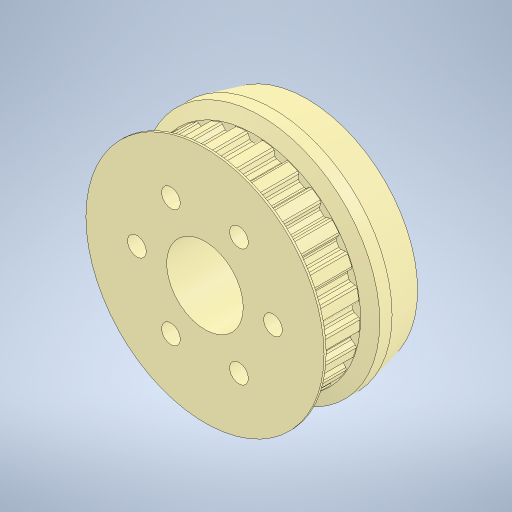
# Autodesk Inventor part: XL Belt Generator
Saved by Autodesk Inventor 2023.4 (Build 274418000, 418)
## iProperties
RuleStatus: InUse
Created: 2022-06-22
Part Number: XL Belt Generator
Material: Nylon 6/6
Document SubType Name: Modeling
Designer: Nathan Cai
Density: 1.13 g/cm^3
Appearance: Nylon 6
Mass: 24.0881 g
Surface Area: 78.8918 cm^2
Volume: 21.3169 cm^3
Author: Nathan Cai
Autodesk Inventor part; units mm, degrees
ref_plane "YZ Plane" through (0, 0, 0) normal (1, 0, 0) x (0, 1, 0)
ref_plane "XZ Plane" through (0, 0, 0) normal (0, 1, 0) x (-1, 0, 0)
ref_plane "XY Plane" through (0, 0, 0) normal (0, 0, 1) x (1, 0, 0)
sketch "Sketch2" plane through (0, 0, 0) normal (0, 0, 1) x (1, 0, 0)
  circle A0 centre (0, 0) radius 20.2127 construction
  circle A1 centre (0, 0) radius 19.6977
  circle A2 centre (0, 0) radius 7.1437
  dimension "Pd" = 40.4254
  dimension "OD" = 39.3954
  dimension "d61" = 14.2875
  constraints: 3 centre point, 3 coincident
  measures "Pd" diameter of A0
  measures "OD" diameter of A1
  measures "d61" diameter of A2
extrude "Extrusion3" add sketch "Sketch2" along normal blind 7.62
sketch "Sketch3" plane through (0, 0, 7.62) normal (0, 0, 1) x (1, 0, 0)
  line L0 (0, 0) -> (0, 19.6977) construction
  circle A0 centre (0, 0) radius 19.6977 projected
  line L1 (0, 0) -> (4.8986, 19.0788) construction
  circle A1 centre (0, 0) radius 18.4277
  line L2 (0.811, 18.6413) -> (1.1735, 19.4185)
  line L3 (1.2841, 19.6558) -> (0, 0) construction
  arc A2 (1.5477, 19.6368) -> (1.1735, 19.4185) centre (1.5179, 19.258) ccw
  arc A3 (0.4572, 18.422) -> (0.811, 18.6413) centre (0.4666, 18.8019) ccw
  circle A4 centre (0, 0) radius 19.6977 projected
  line L4 (-0.811, 18.6413) -> (-1.1735, 19.4185)
  arc A5 (-1.1735, 19.4185) -> (-1.5477, 19.6368) centre (-1.5179, 19.258) ccw
  arc A6 (-0.811, 18.6413) -> (-0.4572, 18.422) centre (-0.4666, 18.8019) ccw
  point P0 (1.807, 18.3389)
  point P1 (1.5477, 19.6368)
  point P2 (-1.5477, 19.6368)
  dimension "d29" = 14.4
  dimension "d30" = 36.8554
  dimension "d31" = 25
  dimension "d33" = 3.738
  dimension "d34" = 0.76
  dimension "d35" = 0.76
  constraints: 14 point on circle, 10 end point, 6 symmetric about line, 5 centre point, 4 tangent, 1 coincident, 1 point on line, 1 vertical, 2 other
  measures "d29" angle of L0 L1
  measures "d30" diameter of A1
  measures "d31" angle of L0 L2
  measures "d33" angle of L0 L3
  measures "d34" diameter of A2
  measures "d35" diameter of A3
extrude "Extrusion4" cut sketch "Sketch3" against normal through all contours A2 L2 A3 A1 A6 L4 A5 A0 picked at (0.0508, 19.2696)
pattern_circular "Circular Pattern2" count 25 over 360 about axis through (0, 0, 0) along (0, 0, 1) of "Extrusion4"
ref_plane "Work Plane1" through (0, 0, 3.81) normal (0, 0, 1) x (1, 0, 0)
sketch "Sketch6" plane through (0, 0, 7.62) normal (0, 0, 1) x (1, 0, 0)
  circle A0 centre (0, 0) radius 22.225
  circle A1 centre (0, 0) radius 7.1437 projected
  dimension "d62" = 44.45
  constraints: 1 centre point, 1 coincident
  measures "d62" diameter of A0
extrude "Extrusion7" add sketch "Sketch6" along normal blind 1.5875
chamfer "Chamfer2" distance 1.1906 distance2 2.3813 1 edges at (-22.225, 0, 7.62) measured on face at (-22.225, 0, 8.12)
mirror "Mirror2" about plane through (0, 0, 3.81) normal (0, 0, 1) of "Extrusion7", "Chamfer2"
thicken "Thicken3" operation add thickness 1.905 both sides no extend neighbours no toward (0, 0, -1) faces at (16.9134, -2.3428, -1.5875)
thicken "Thicken4" operation add thickness 6.35 both sides no extend neighbours no toward (0, 0, -1) faces at (16.9134, -2.3428, -3.4925)
chamfer "Chamfer3" distance 6.35 distance2 1.5875 1 edges at (-22.225, 0, -9.8425) measured on face at (-22.225, 0, -9.3425)
sketch "Sketch7" plane through (0, 0, -9.8425) normal (0, 0, -1) x (-1, 0, 0)
  circle A0 centre (0, 0) radius 12.7 construction
  line L0 (0, 0) -> (12.7, 0) construction
  circle A1 centre (12.7, 0) radius 1.7526
  circle A2 centre (6.35, 10.9985) radius 1.7526
  circle A3 centre (-6.35, 10.9985) radius 1.7526
  circle A4 centre (-12.7, 0) radius 1.7526
  circle A5 centre (-6.35, -10.9985) radius 1.7526
  circle A6 centre (6.35, -10.9985) radius 1.7526
  dimension "d75" = 25.4
  dimension "d76" = 3.5052
  dimension "d79" = 360
  constraints: 6 centre point, 2 coincident, 2 end point, 1 horizontal, 1 horizontal alignment, 15 other
  measures "d76" diameter of A1
extrude "Extrusion8" cut sketch "Sketch7" against normal through all
equation "\"pitch\" = 5.08"
equation "\"width\" = 7.62"
equation "\"T_angle\" = 50deg"
equation "\"T_ht\" = 1.27"
equation "\"r1\" = 0.38"
equation "\"r2\" = 0.38"
equation "\"T_hs\" = 2.3"
equation "\"T_s\" = 2.57"
equation "\"Bore\" = 14.2875"
body "Solid3"
